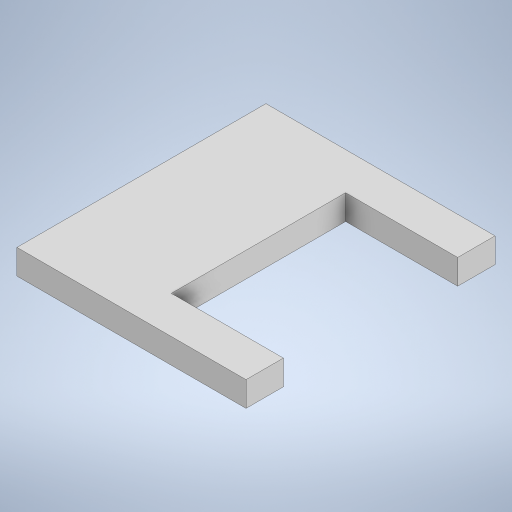
# Autodesk Inventor part: Poperechnik
Saved by Autodesk Inventor 2024 (Build 280153000, 153)
## iProperties
Created: 2023-08-21
Part Number: Poperechnik
Material: Generic
Document SubType Name: Modeling
Designer: KirikDK
Density: 1 g/cm^3
Appearance: Default
Author: KirikDK
Autodesk Inventor part; units mm, degrees
ref_plane "YZ Plane" through (0, 0, 0) normal (1, 0, 0) x (0, 1, 0)
ref_plane "XZ Plane" through (0, 0, 0) normal (0, 1, 0) x (-1, 0, 0)
ref_plane "XY Plane" through (0, 0, 0) normal (0, 0, 1) x (1, 0, 0)
sketch "Sketch1" plane through (0, 0, 0) normal (0, 1, 0) x (-1, 0, 0)
  point P0 (0, 0)
sketch "Sketch2" plane through (0, 0, 0) normal (0, 1, 0) x (-1, 0, 0)
  line L0 (26.6667, 55.5556) -> (-65.3333, 55.5556)
  line L1 (-65.3333, 55.5556) -> (-65.3333, -44.4444)
  line L2 (-65.3333, -44.4444) -> (26.6667, -44.4444)
  line L3 (26.6667, -44.4444) -> (26.6667, 55.5556)
  point P0 (0, 0)
  dimension "d0" = 100
  dimension "d1" = 92
  constraints: 8 end point, 2 parallel, 1 horizontal, 1 perpendicular
  measures "d0" distance of L2.end L0.start
  measures "d1" distance of L1.end L2.end
extrude "Extrusion1" add sketch "Sketch2" along normal blind 10
sketch "Sketch3" plane through (0, 10, 0) normal (0, 1, 0) x (1, 0, 0)
  line L0 (65.3333, -55.5556) -> (65.3333, 44.4444) projected
  line L1 (65.3333, 29.4444) -> (20.3333, 29.4444)
  line L2 (20.3333, 29.4444) -> (20.3333, -40.5556)
  line L3 (20.3333, -40.5556) -> (65.3333, -40.5556)
  line L4 (65.3333, -40.5556) -> (65.3333, 29.4444)
  line L5 (65.3333, 44.4444) -> (-26.6667, 44.4444) projected
  line L6 (-26.6667, -55.5556) -> (65.3333, -55.5556) projected
  point P0 (0, 0)
  point P1 (65.3333, -40.5556)
  dimension "d4" = 70
  dimension "d5" = 15
  dimension "d6" = 15
  dimension "d7" = 45
  constraints: 8 end point, 2 parallel, 1 horizontal, 1 perpendicular, 1 point on line
  measures "d4" distance of L1.end L2.end
  measures "d5" distance between parallel lines of L5 L1
  measures "d6" distance between parallel lines of L6 L3
  measures "d7" distance of L2.end L3.end
extrude "Extrusion2" cut sketch "Sketch3" along normal mid plane 100
body "Solid1"
